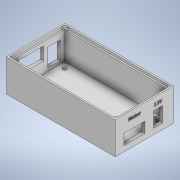
# Autodesk Inventor part: Caixa plaquinha valvulav2
Saved by Autodesk Inventor 2020 (Build 240168000, 168)
## iProperties
Created: 2022-10-16
Part Number: Caixa plaquinha valvulav2
Material: Genérico
Document SubType Name: Modeling
Designer: Gabriel
Density: 1 g/cm^3
Appearance: Padrão
Author: Gabriel
Autodesk Inventor part; units mm, degrees
ref_plane "YZ Plane" through (0, 0, 0) normal (1, 0, 0) x (0, 1, 0)
ref_plane "XZ Plane" through (0, 0, 0) normal (0, 1, 0) x (-1, 0, 0)
ref_plane "XY Plane" through (0, 0, 0) normal (0, 0, 1) x (1, 0, 0)
sketch "Esboço1" plane through (0, 0, 0) normal (0, 1, 0) x (-1, 0, 0)
  line L0 (62.5795, 27.2159) -> (-45.4205, 27.2159)
  line L1 (-45.4205, 27.2159) -> (-45.4205, -30.7841)
  line L2 (-45.4205, -30.7841) -> (62.5795, -30.7841)
  line L3 (62.5795, -30.7841) -> (62.5795, 27.2159)
  point P0 (0, 0)
  dimension "d0" = 58
  dimension "d1" = 108
  constraints: 8 end point, 2 parallel, 1 horizontal, 1 perpendicular
  measures "d0" distance between parallel lines of L2 L0
  measures "d1" distance of L1.end L2.end
extrude "Extrusão1" add sketch "Esboço1" along normal blind 32
sketch "Esboço2" plane through (0, 32, 0) normal (0, 1, 0) x (1, 0, 0)
  line L0 (-59.5795, 27.7841) -> (42.4205, 27.7841)
  line L1 (42.4205, 27.7841) -> (42.4205, -24.2159)
  line L2 (42.4205, -24.2159) -> (-59.5795, -24.2159)
  line L3 (-59.5795, -24.2159) -> (-59.5795, 27.7841)
  line L4 (-62.5795, 30.7841) -> (-62.5795, -27.2159) projected
  line L5 (45.4205, 30.7841) -> (-62.5795, 30.7841) projected
  point P0 (0, 0)
  dimension "d4" = 3
  dimension "d5" = 102
  dimension "d6" = 3
  dimension "d7" = 52
  constraints: 8 end point, 2 parallel, 1 horizontal, 1 perpendicular
  measures "d4" distance between parallel lines of L4 L3
  measures "d5" distance between parallel lines of L1 L3
  measures "d6" distance between parallel lines of L5 L0
  measures "d7" distance between parallel lines of L0 L2
extrude "Extrusão2" cut sketch "Esboço2" against normal blind 30
sketch "Esboço4" plane through (0, 32, 0) normal (0, 1, 0) x (1, 0, 0)
  line L0 (-61.0795, 29.2841) -> (43.9205, 29.2841)
  line L1 (43.9205, 29.2841) -> (43.9205, -25.7159)
  line L2 (43.9205, -25.7159) -> (-61.0795, -25.7159)
  line L3 (-61.0795, -25.7159) -> (-61.0795, 29.2841)
  line L4 (45.4205, 30.7841) -> (-62.5795, 30.7841) projected
  line L5 (-62.5795, 30.7841) -> (-62.5795, -27.2159) projected
  line L6 (-62.5795, -27.2159) -> (45.4205, -27.2159) projected
  line L7 (45.4205, -27.2159) -> (45.4205, 30.7841) projected
  point P0 (0, 0)
  dimension "d10" = 1.5
  dimension "d11" = 1.5
  dimension "d12" = 1.5
  dimension "d13" = 1.5
  constraints: 8 end point, 2 parallel, 1 horizontal, 1 perpendicular
  measures "d10" distance between parallel lines of L4 L0
  measures "d11" distance between parallel lines of L5 L3
  measures "d12" distance between parallel lines of L6 L2
  measures "d13" distance between parallel lines of L7 L1
extrude "Extrusão3" cut sketch "Esboço4" against normal blind 2.5 contours L0 L1 L2 L3
sketch "Esboço5" plane through (42.4205, 2, -27.7841) normal (-1, 0, 0) x (0, 0, 1)
  line L0 (0, 0) -> (52, 0) projected
  line L1 (8.1, 3.75) -> (17.1, 3.75)
  line L2 (17.1, 3.75) -> (17.1, 18.75)
  line L3 (17.1, 18.75) -> (8.1, 18.75)
  line L4 (8.1, 18.75) -> (8.1, 3.75)
  line L5 (46.3, 3.5) -> (25.6, 3.5)
  line L6 (25.6, 3.5) -> (25.6, 14)
  line L7 (25.6, 14) -> (46.3, 14)
  line L8 (46.3, 14) -> (46.3, 3.5)
  line L9 (52, 27.5) -> (0, 27.5) projected
  point P0 (27.7841, -2)
  point P1 (25.6, 0)
  point P2 (17.1, 0)
  dimension "d17" = 9
  dimension "d20" = 20.7
  dimension "d23" = 8.5
  dimension "d24" = 8.1
  dimension "d25" = 5.7
  dimension "d55" = 3.75
  dimension "d56" = 15
  dimension "d57" = 3.5
  dimension "d58" = 10.5
  constraints: 16 end point, 4 parallel, 2 horizontal, 2 perpendicular
  measures "d17" distance between parallel lines of L2 L4
  measures "d20" distance between parallel lines of L6 L8
  measures "d23" distance between parallel lines of L6 L2
  measures "d24" distance from line of L9.end L4
  measures "d25" distance from line of L9.start L8
  measures "d55" distance between parallel lines of L1 L0
  measures "d56" distance between parallel lines of L3 L1
  measures "d57" distance between parallel lines of L0 L5
  measures "d58" distance between parallel lines of L7 L5
extrude "Extrusão4" cut sketch "Esboço5" against normal blind 5
sketch "Esboço6" plane through (0, 2, 0) normal (0, 1, 0) x (1, 0, 0)
  line L0 (45.4205, 2.1841) -> (45.4205, -18.5159) projected
  line L1 (42.4205, 27.7841) -> (42.4205, -24.2159) projected
  line L2 (45.4205, -18.5159) -> (42.4205, -18.5159)
  line L3 (42.4205, -18.5159) -> (42.4205, 2.1841)
  line L4 (42.4205, 2.1841) -> (45.4205, 2.1841)
  line L5 (45.4205, 2.1841) -> (45.4205, -18.5159)
  line L6 (45.4205, 19.6841) -> (45.4205, 10.6841) projected
  line L7 (45.4205, 19.6841) -> (42.4205, 19.6841)
  line L8 (42.4205, 19.6841) -> (42.4205, 10.6841)
  line L9 (42.4205, 10.6841) -> (45.4205, 10.6841)
  line L10 (45.4205, 10.6841) -> (45.4205, 19.6841)
  point P0 (0, 0)
  point P1 (42.4205, 10.6841)
  constraints: 16 end point, 4 parallel, 2 horizontal, 2 perpendicular, 1 point on line
extrude "Extrusão5" add sketch "Esboço6" along normal blind 1
sketch "Esboço7" plane through (-59.5795, 2, 24.2159) normal (1, 0, 0) x (0, 0, -1)
  line L0 (47.5, 3) -> (35, 3)
  line L1 (35, 3) -> (35, 21)
  line L2 (35, 21) -> (47.5, 21)
  line L3 (47.5, 21) -> (47.5, 3)
  line L4 (6, 11) -> (31, 11)
  line L5 (31, 11) -> (31, 24)
  line L6 (31, 24) -> (6, 24)
  line L7 (6, 24) -> (6, 11)
  line L8 (0, 0) -> (52, 0) projected
  point P0 (24.2159, -2)
  point P1 (52, 27.5)
  point P2 (0, 27.5)
  dimension "d31" = 4.5
  dimension "d32" = 12.5
  dimension "d33" = 6
  dimension "d34" = 25
  dimension "d35" = 13
  dimension "d36" = 11
  dimension "d39" = 18
  dimension "d59" = 3
  constraints: 16 end point, 4 parallel, 2 horizontal, 2 perpendicular
  measures "d31" distance from line of L3 point (52, 27.5)
  measures "d32" distance between parallel lines of L3 L1
  measures "d33" distance from line of point (0, 27.5) L7
  measures "d34" distance between parallel lines of L5 L7
  measures "d35" distance between parallel lines of L6 L4
  measures "d36" distance between parallel lines of L8 L4
  measures "d39" distance between parallel lines of L0 L2
  measures "d59" distance between parallel lines of L8 L0
extrude "Extrusão6" cut sketch "Esboço7" against normal blind 5
sketch "Esboço9" plane through (0, 2, 0) normal (0, 1, 0) x (1, 0, 0)
  line L0 (42.4205, -24.2159) -> (-59.5795, -24.2159) projected
  line L1 (5.9205, -24.2159) -> (10.9205, -24.2159)
  line L2 (10.9205, -24.2159) -> (10.9205, -27.2159)
  line L3 (10.9205, -27.2159) -> (5.9205, -27.2159)
  line L4 (5.9205, -27.2159) -> (5.9205, -24.2159)
  line L5 (10.9205, -27.2159) -> (5.9205, -27.2159) projected
  point P0 (0, 0)
  dimension "d50" = 0
  constraints: 8 end point, 2 parallel, 1 horizontal, 1 perpendicular
  measures "d50" distance between parallel lines of L5 L3
extrude "Extrusão8" add sketch "Esboço9" along normal blind 1
sketch "Esboço10" plane through (45.4205, 0, 27.2159) normal (1, 0, 0) x (0, 0, -1)
  line L0 (36.0799, 28.5533) -> (48.8276, 28.5533) construction
  line L1 (48.8276, 28.5533) -> (48.8276, 22.0035) construction
  line L2 (48.8276, 22.0035) -> (36.0799, 22.0035) construction
  line L3 (36.0799, 22.0035) -> (36.0799, 28.5533) construction
  line L4 (13.7499, 26.9393) -> (24.4451, 26.9393) construction
  line L5 (24.4451, 26.9393) -> (24.4451, 23.827) construction
  line L6 (24.4451, 23.827) -> (13.7499, 23.827) construction
  line L7 (13.7499, 23.827) -> (13.7499, 26.9393) construction
  line L8 (16.286, 23.8893) -> (15.5247, 23.8893)
  line L9 (15.5247, 23.8893) -> (15.5247, 25.9111)
  line L10 (15.5247, 25.9111) -> (14.9711, 24.606)
  line L11 (14.9711, 24.606) -> (14.4471, 24.606)
  line L12 (14.4471, 24.606) -> (13.8935, 25.9111)
  line L13 (13.8935, 25.9111) -> (13.8935, 23.8893)
  line L14 (13.8935, 23.8893) -> (13.1717, 23.8893)
  line L15 (13.1717, 23.8893) -> (13.1717, 26.9393)
  line L16 (13.1717, 26.9393) -> (14.0541, 26.9393)
  line L17 (14.0541, 26.9393) -> (14.7313, 25.434)
  line L18 (14.7313, 25.434) -> (15.4036, 26.9393)
  line L19 (15.4036, 26.9393) -> (16.286, 26.9393)
  line L20 (16.286, 26.9393) -> (16.286, 23.8893)
  spline S0 degree 2 poles (19.0839, 25.0386) (19.0839, 24.4701) (18.4635, 23.8176) (17.8975, 23.8176) knots 0 0 0 1 2 2 2
  spline S1 degree 2 poles (17.8975, 23.8176) (17.334, 23.8176) (16.7087, 24.4701) (16.7087, 25.0386) knots 0 0 0 1 2 2 2
  spline S2 degree 2 poles (16.7087, 25.0386) (16.7087, 25.612) (17.334, 26.262) (17.8975, 26.262) knots 0 0 0 1 2 2 2
  spline S3 degree 2 poles (17.8975, 26.262) (18.461, 26.262) (19.0839, 25.6095) (19.0839, 25.0386) knots 0 0 0 1 2 2 2
  spline S4 degree 2 poles (18.3498, 25.0336) (18.3498, 25.2388) (18.2831, 25.5131) (18.2238, 25.5947) knots 0 0 0 1 2 2 2
  spline S5 degree 2 poles (18.2238, 25.5947) (18.1595, 25.6812) (17.9989, 25.7479) (17.8975, 25.7479) knots 0 0 0 1 2 2 2
  spline S6 degree 2 poles (17.8975, 25.7479) (17.7986, 25.7479) (17.6429, 25.6886) (17.5787, 25.6046) knots 0 0 0 1 2 2 2
  spline S7 degree 2 poles (17.5787, 25.6046) (17.5169, 25.5255) (17.4427, 25.2462) (17.4427, 25.0336) knots 0 0 0 1 2 2 2
  spline S8 degree 2 poles (17.4427, 25.0336) (17.4427, 24.8235) (17.5119, 24.564) (17.5688, 24.4849) knots 0 0 0 1 2 2 2
  spline S9 degree 2 poles (17.5688, 24.4849) (17.6256, 24.4058) (17.7986, 24.3317) (17.9025, 24.3317) knots 0 0 0 1 2 2 2
  spline S10 degree 2 poles (17.9025, 24.3317) (17.989, 24.3317) (18.1669, 24.4058) (18.2213, 24.48) knots 0 0 0 1 2 2 2
  spline S11 degree 2 poles (18.2213, 24.48) (18.2831, 24.5665) (18.3498, 24.8161) (18.3498, 25.0336) knots 0 0 0 1 2 2 2
  spline S12 degree 2 poles (20.3444, 23.8448) (19.907, 23.8448) (19.5065, 24.2056) (19.5065, 24.6159) knots 0 0 0 1 2 2 2
  line L21 (19.5065, 24.6159) -> (19.5065, 25.6911)
  line L22 (19.5065, 25.6911) -> (19.2322, 25.6911)
  line L23 (19.2322, 25.6911) -> (19.2322, 26.1904)
  line L24 (19.2322, 26.1904) -> (19.5065, 26.1904)
  line L25 (19.5065, 26.1904) -> (19.5065, 26.8478)
  line L26 (19.5065, 26.8478) -> (20.2233, 26.8478)
  line L27 (20.2233, 26.8478) -> (20.2233, 26.1904)
  line L28 (20.2233, 26.1904) -> (20.9154, 26.1904)
  line L29 (20.9154, 26.1904) -> (20.9154, 25.6911)
  line L30 (20.9154, 25.6911) -> (20.2233, 25.6911)
  line L31 (20.2233, 25.6911) -> (20.2233, 24.873)
  spline S13 degree 2 poles (20.2233, 24.873) (20.2233, 24.7519) (20.2283, 24.5714) (20.2579, 24.4998) knots 0 0 0 1 2 2 2
  spline S14 degree 2 poles (20.2579, 24.4998) (20.2876, 24.4281) (20.4334, 24.344) (20.5718, 24.344) knots 0 0 0 1 2 2 2
  spline S15 degree 2 poles (20.5718, 24.344) (20.6311, 24.344) (20.8165, 24.3935) (20.8536, 24.4132) knots 0 0 0 1 2 2 2
  line L32 (20.8536, 24.4132) -> (20.9154, 24.4132)
  line L33 (20.9154, 24.4132) -> (20.9154, 23.909)
  spline S16 degree 2 poles (20.9154, 23.909) (20.7992, 23.8794) (20.5372, 23.8448) (20.3444, 23.8448) knots 0 0 0 1 2 2 2
  spline S17 degree 2 poles (23.4142, 25.0386) (23.4142, 24.4701) (22.7938, 23.8176) (22.2278, 23.8176) knots 0 0 0 1 2 2 2
  spline S18 degree 2 poles (22.2278, 23.8176) (21.6643, 23.8176) (21.039, 24.4701) (21.039, 25.0386) knots 0 0 0 1 2 2 2
  spline S19 degree 2 poles (21.039, 25.0386) (21.039, 25.612) (21.6643, 26.262) (22.2278, 26.262) knots 0 0 0 1 2 2 2
  spline S20 degree 2 poles (22.2278, 26.262) (22.7914, 26.262) (23.4142, 25.6095) (23.4142, 25.0386) knots 0 0 0 1 2 2 2
  spline S21 degree 2 poles (22.6801, 25.0336) (22.6801, 25.2388) (22.6134, 25.5131) (22.5541, 25.5947) knots 0 0 0 1 2 2 2
  spline S22 degree 2 poles (22.5541, 25.5947) (22.4898, 25.6812) (22.3292, 25.7479) (22.2278, 25.7479) knots 0 0 0 1 2 2 2
  spline S23 degree 2 poles (22.2278, 25.7479) (22.129, 25.7479) (21.9732, 25.6886) (21.909, 25.6046) knots 0 0 0 1 2 2 2
  spline S24 degree 2 poles (21.909, 25.6046) (21.8472, 25.5255) (21.773, 25.2462) (21.773, 25.0336) knots 0 0 0 1 2 2 2
  spline S25 degree 2 poles (21.773, 25.0336) (21.773, 24.8235) (21.8422, 24.564) (21.8991, 24.4849) knots 0 0 0 1 2 2 2
  spline S26 degree 2 poles (21.8991, 24.4849) (21.9559, 24.4058) (22.129, 24.3317) (22.2328, 24.3317) knots 0 0 0 1 2 2 2
  spline S27 degree 2 poles (22.2328, 24.3317) (22.3193, 24.3317) (22.4972, 24.4058) (22.5516, 24.48) knots 0 0 0 1 2 2 2
  spline S28 degree 2 poles (22.5516, 24.48) (22.6134, 24.5665) (22.6801, 24.8161) (22.6801, 25.0336) knots 0 0 0 1 2 2 2
  line L34 (25.3396, 25.5106) -> (25.2803, 25.5106)
  spline S29 degree 2 poles (25.2803, 25.5106) (25.2383, 25.5255) (25.0826, 25.5403) (24.9886, 25.5403) knots 0 0 0 1 2 2 2
  spline S30 degree 2 poles (24.9886, 25.5403) (24.8774, 25.5403) (24.6278, 25.4736) (24.5116, 25.4291) knots 0 0 0 1 2 2 2
  line L35 (24.5116, 25.4291) -> (24.5116, 23.8893)
  line L36 (24.5116, 23.8893) -> (23.7948, 23.8893)
  line L37 (23.7948, 23.8893) -> (23.7948, 26.1904)
  line L38 (23.7948, 26.1904) -> (24.5116, 26.1904)
  line L39 (24.5116, 26.1904) -> (24.5116, 25.8592)
  spline S31 degree 2 poles (24.5116, 25.8592) (24.561, 25.9036) (24.7341, 26.0421) (24.8057, 26.0841) knots 0 0 0 1 2 2 2
  spline S32 degree 2 poles (24.8057, 26.0841) (24.8848, 26.131) (25.0924, 26.1978) (25.1839, 26.1978) knots 0 0 0 1 2 2 2
  spline S33 degree 2 poles (25.1839, 26.1978) (25.2185, 26.1978) (25.305, 26.1928) (25.3396, 26.1904) knots 0 0 0 1 2 2 2
  line L40 (25.3396, 26.1904) -> (25.3396, 25.5106)
  line L41 (40.7496, 23.7237) -> (38.7352, 23.7237)
  line L42 (38.7352, 23.7237) -> (38.7352, 24.2551)
  line L43 (38.7352, 24.2551) -> (39.3778, 24.2551)
  line L44 (39.3778, 24.2551) -> (39.3778, 25.8691)
  line L45 (39.3778, 25.8691) -> (38.7352, 25.8691)
  line L46 (38.7352, 25.8691) -> (38.7352, 26.3659)
  spline S34 degree 2 poles (38.7352, 26.3659) (38.8761, 26.3659) (39.1554, 26.403) (39.2394, 26.4425) knots 0 0 0 1 2 2 2
  spline S35 degree 2 poles (39.2394, 26.4425) (39.3358, 26.492) (39.4445, 26.6576) (39.4544, 26.7811) knots 0 0 0 1 2 2 2
  line L47 (39.4544, 26.7811) -> (40.1218, 26.7811)
  line L48 (40.1218, 26.7811) -> (40.1218, 24.2551)
  line L49 (40.1218, 24.2551) -> (40.7496, 24.2551)
  line L50 (40.7496, 24.2551) -> (40.7496, 23.7237)
  line L51 (43.5573, 23.7237) -> (41.3156, 23.7237)
  line L52 (41.3156, 23.7237) -> (41.3156, 24.2205)
  spline S36 degree 2 poles (41.3156, 24.2205) (41.5998, 24.4479) (42.0546, 24.8483) (42.2251, 25.0288) knots 0 0 0 1 2 2 2
  spline S37 degree 2 poles (42.2251, 25.0288) (42.45, 25.2636) (42.6502, 25.6219) (42.6502, 25.8098) knots 0 0 0 1 2 2 2
  spline S38 degree 2 poles (42.6502, 25.8098) (42.6502, 26.0224) (42.3957, 26.2497) (42.1683, 26.2497) knots 0 0 0 1 2 2 2
  spline S39 degree 2 poles (42.1683, 26.2497) (42.0521, 26.2497) (41.8445, 26.1929) (41.7382, 26.1484) knots 0 0 0 1 2 2 2
  spline S40 degree 2 poles (41.7382, 26.1484) (41.6344, 26.1014) (41.4861, 26.0026) (41.449, 25.9779) knots 0 0 0 1 2 2 2
  line L53 (41.449, 25.9779) -> (41.3897, 25.9779)
  line L54 (41.3897, 25.9779) -> (41.3897, 26.6427)
  spline S41 degree 2 poles (41.3897, 26.6427) (41.5182, 26.7045) (42.0669, 26.833) (42.3215, 26.833) knots 0 0 0 1 2 2 2
  spline S42 degree 2 poles (42.3215, 26.833) (42.8653, 26.833) (43.4239, 26.3486) (43.4239, 25.9111) knots 0 0 0 1 2 2 2
  spline S43 degree 2 poles (43.4239, 25.9111) (43.4239, 25.6417) (43.1693, 25.1227) (42.8752, 24.8261) knots 0 0 0 1 2 2 2
  spline S44 degree 2 poles (42.8752, 24.8261) (42.6898, 24.6432) (42.3413, 24.3589) (42.2647, 24.2996) knots 0 0 0 1 2 2 2
  line L55 (42.2647, 24.2996) -> (43.5573, 24.2996)
  line L56 (43.5573, 24.2996) -> (43.5573, 23.7237)
  line L57 (46.5406, 26.7737) -> (45.4926, 23.7237)
  line L58 (45.4926, 23.7237) -> (44.6943, 23.7237)
  line L59 (44.6943, 23.7237) -> (43.6463, 26.7737)
  line L60 (43.6463, 26.7737) -> (44.4397, 26.7737)
  line L61 (44.4397, 26.7737) -> (45.1046, 24.705)
  line L62 (45.1046, 24.705) -> (45.767, 26.7737)
  line L63 (45.767, 26.7737) -> (46.5406, 26.7737)
  point P0 (27.2159, 0)
  constraints: 4 other
extrude "Extrusão9" cut sketch "Esboço10" against normal blind 0.8
sketch "Esboço11" plane through (-62.5795, 0, -30.7841) normal (-1, 0, 0) x (0, 0, 1)
  line L0 (32.154, 11.2221) -> (40.856, 11.2221) construction
  line L1 (40.856, 11.2221) -> (40.856, 8.0726) construction
  line L2 (40.856, 8.0726) -> (32.154, 8.0726) construction
  line L3 (32.154, 8.0726) -> (32.154, 11.2221) construction
  line L4 (7.8779, 28.5473) -> (19.6465, 28.5473) construction
  line L5 (19.6465, 28.5473) -> (19.6465, 24.5765) construction
  line L6 (19.6465, 24.5765) -> (7.8779, 24.5765) construction
  line L7 (7.8779, 24.5765) -> (7.8779, 28.5473) construction
  line L8 (8.874, 26.9175) -> (7.8103, 26.9175)
  line L9 (7.8103, 26.9175) -> (7.8103, 27.2265)
  line L10 (7.8103, 27.2265) -> (8.874, 27.2265)
  line L11 (8.874, 27.2265) -> (8.874, 26.9175)
  spline S0 degree 2 poles (12.5502, 26.6874) (12.5502, 26.5381) (12.4113, 26.2478) (12.2869, 26.1483) knots 0 0 0 1 2 2 2
  spline S1 degree 2 poles (12.2869, 26.1483) (12.1501, 26.0384) (11.7872, 25.916) (11.5322, 25.916) knots 0 0 0 1 2 2 2
  spline S2 degree 2 poles (11.5322, 25.916) (11.2564, 25.916) (10.8168, 26.0176) (10.5908, 26.1192) knots 0 0 0 1 2 2 2
  line L12 (10.5908, 26.1192) -> (10.5908, 26.5422)
  line L13 (10.5908, 26.5422) -> (10.6157, 26.5422)
  spline S3 degree 2 poles (10.6157, 26.5422) (10.8085, 26.3826) (11.3124, 26.2084) (11.5363, 26.2084) knots 0 0 0 1 2 2 2
  spline S4 degree 2 poles (11.5363, 26.2084) (11.8494, 26.2084) (12.1998, 26.4427) (12.1998, 26.6397) knots 0 0 0 1 2 2 2
  spline S5 degree 2 poles (12.1998, 26.6397) (12.1998, 26.8076) (12.0339, 26.9673) (11.8639, 27.0129) knots 0 0 0 1 2 2 2
  spline S6 degree 2 poles (11.8639, 27.0129) (11.7374, 27.0461) (11.4368, 27.0917) (11.2709, 27.1249) knots 0 0 0 1 2 2 2
  spline S7 degree 2 poles (11.2709, 27.1249) (10.9309, 27.1974) (10.6053, 27.5437) (10.6053, 27.8216) knots 0 0 0 1 2 2 2
  spline S8 degree 2 poles (10.6053, 27.8216) (10.6053, 28.1388) (11.1444, 28.5473) (11.5612, 28.5473) knots 0 0 0 1 2 2 2
  spline S9 degree 2 poles (11.5612, 28.5473) (11.8287, 28.5473) (12.2765, 28.4457) (12.4486, 28.369) knots 0 0 0 1 2 2 2
  line L14 (12.4486, 28.369) -> (12.4486, 27.9708)
  line L15 (12.4486, 27.9708) -> (12.4238, 27.9708)
  spline S10 degree 2 poles (12.4238, 27.9708) (12.2786, 28.0932) (11.8059, 28.2549) (11.5571, 28.2549) knots 0 0 0 1 2 2 2
  spline S11 degree 2 poles (11.5571, 28.2549) (11.2854, 28.2549) (10.9557, 28.031) (10.9557, 27.8527) knots 0 0 0 1 2 2 2
  spline S12 degree 2 poles (10.9557, 27.8527) (10.9557, 27.6951) (11.1195, 27.5147) (11.3269, 27.467) knots 0 0 0 1 2 2 2
  spline S13 degree 2 poles (11.3269, 27.467) (11.4368, 27.4421) (11.839, 27.3737) (11.98, 27.3384) knots 0 0 0 1 2 2 2
  spline S14 degree 2 poles (11.98, 27.3384) (12.2641, 27.2638) (12.5502, 26.959) (12.5502, 26.6874) knots 0 0 0 1 2 2 2
  line L16 (13.3921, 25.9617) -> (13.0707, 25.9617)
  line L17 (13.0707, 25.9617) -> (13.0707, 27.8672)
  line L18 (13.0707, 27.8672) -> (13.3921, 27.8672)
  line L19 (13.3921, 27.8672) -> (13.3921, 25.9617)
  line L20 (13.4128, 28.1865) -> (13.0499, 28.1865)
  line L21 (13.0499, 28.1865) -> (13.0499, 28.5182)
  line L22 (13.0499, 28.5182) -> (13.4128, 28.5182)
  line L23 (13.4128, 28.5182) -> (13.4128, 28.1865)
  spline S15 degree 2 poles (15.5734, 26.1794) (15.5734, 25.6942) (15.1338, 25.2401) (14.6755, 25.2401) knots 0 0 0 1 2 2 2
  spline S16 degree 2 poles (14.6755, 25.2401) (14.5242, 25.2401) (14.236, 25.2836) (14.095, 25.321) knots 0 0 0 1 2 2 2
  line L24 (14.095, 25.321) -> (14.095, 25.6486)
  line L25 (14.095, 25.6486) -> (14.1116, 25.6486)
  spline S17 degree 2 poles (14.1116, 25.6486) (14.1904, 25.6175) (14.5325, 25.5283) (14.7025, 25.5283) knots 0 0 0 1 2 2 2
  spline S18 degree 2 poles (14.7025, 25.5283) (14.8663, 25.5283) (15.0819, 25.6071) (15.1421, 25.6755) knots 0 0 0 1 2 2 2
  spline S19 degree 2 poles (15.1421, 25.6755) (15.2001, 25.7419) (15.252, 25.9306) (15.252, 26.0467) knots 0 0 0 1 2 2 2
  line L26 (15.252, 26.0467) -> (15.252, 26.2188)
  spline S20 degree 2 poles (15.252, 26.2188) (15.1068, 26.1026) (14.8435, 25.9886) (14.6382, 25.9886) knots 0 0 0 1 2 2 2
  spline S21 degree 2 poles (14.6382, 25.9886) (14.2961, 25.9886) (13.8959, 26.4821) (13.8959, 26.932) knots 0 0 0 1 2 2 2
  spline S22 degree 2 poles (13.8959, 26.932) (13.8959, 27.1788) (14.0348, 27.5354) (14.153, 27.664) knots 0 0 0 1 2 2 2
  spline S23 degree 2 poles (14.153, 27.664) (14.265, 27.7863) (14.5822, 27.9211) (14.7378, 27.9211) knots 0 0 0 1 2 2 2
  spline S24 degree 2 poles (14.7378, 27.9211) (14.9036, 27.9211) (15.1276, 27.8547) (15.252, 27.7863) knots 0 0 0 1 2 2 2
  line L27 (15.252, 27.7863) -> (15.2727, 27.8672)
  line L28 (15.2727, 27.8672) -> (15.5734, 27.8672)
  line L29 (15.5734, 27.8672) -> (15.5734, 26.1794)
  line L30 (15.252, 26.4842) -> (15.252, 27.525)
  spline S25 degree 2 poles (15.252, 27.525) (15.1234, 27.5831) (14.9036, 27.6329) (14.7958, 27.6329) knots 0 0 0 1 2 2 2
  spline S26 degree 2 poles (14.7958, 27.6329) (14.5304, 27.6329) (14.2277, 27.2762) (14.2277, 26.9383) knots 0 0 0 1 2 2 2
  spline S27 degree 2 poles (14.2277, 26.9383) (14.2277, 26.6169) (14.4537, 26.2851) (14.7129, 26.2851) knots 0 0 0 1 2 2 2
  spline S28 degree 2 poles (14.7129, 26.2851) (14.8539, 26.2851) (15.1338, 26.3929) (15.252, 26.4842) knots 0 0 0 1 2 2 2
  line L31 (19.6166, 26.9362) -> (18.6877, 26.9362)
  line L32 (18.6877, 26.9362) -> (18.6877, 26.0073)
  line L33 (18.6877, 26.0073) -> (18.4036, 26.0073)
  line L34 (18.4036, 26.0073) -> (18.4036, 26.9362)
  line L35 (18.4036, 26.9362) -> (17.4747, 26.9362)
  line L36 (17.4747, 26.9362) -> (17.4747, 27.2099)
  line L37 (17.4747, 27.2099) -> (18.4036, 27.2099)
  line L38 (18.4036, 27.2099) -> (18.4036, 28.1388)
  line L39 (18.4036, 28.1388) -> (18.6877, 28.1388)
  line L40 (18.6877, 28.1388) -> (18.6877, 27.2099)
  line L41 (18.6877, 27.2099) -> (19.6166, 27.2099)
  line L42 (19.6166, 27.2099) -> (19.6166, 26.9362)
  spline S29 degree 2 poles (33.738, 8.0535) (33.1226, 8.0535) (32.4602, 8.6467) (32.4602, 9.2201) knots 0 0 0 1 2 2 2
  line L43 (32.4602, 9.2201) -> (32.4602, 11.1677)
  line L44 (32.4602, 11.1677) -> (33.2264, 11.1677)
  line L45 (33.2264, 11.1677) -> (33.2264, 9.2646)
  spline S30 degree 2 poles (33.2264, 9.2646) (33.2264, 8.9457) (33.4661, 8.6343) (33.738, 8.6343) knots 0 0 0 1 2 2 2
  spline S31 degree 2 poles (33.738, 8.6343) (34.0025, 8.6343) (34.2496, 8.9334) (34.2496, 9.2646) knots 0 0 0 1 2 2 2
  line L46 (34.2496, 9.2646) -> (34.2496, 11.1677)
  line L47 (34.2496, 11.1677) -> (35.0158, 11.1677)
  line L48 (35.0158, 11.1677) -> (35.0158, 9.2225)
  spline S32 degree 2 poles (35.0158, 9.2225) (35.0158, 8.659) (34.3708, 8.0535) (33.738, 8.0535) knots 0 0 0 1 2 2 2
  spline S33 degree 2 poles (36.5458, 8.0634) (36.1948, 8.0634) (35.6659, 8.1993) (35.4385, 8.2982) knots 0 0 0 1 2 2 2
  line L49 (35.4385, 8.2982) -> (35.4385, 9.0248)
  line L50 (35.4385, 9.0248) -> (35.5077, 9.0248)
  spline S34 degree 2 poles (35.5077, 9.0248) (35.7376, 8.8296) (36.2887, 8.6195) (36.5483, 8.6195) knots 0 0 0 1 2 2 2
  spline S35 degree 2 poles (36.5483, 8.6195) (36.615, 8.6195) (36.83, 8.6491) (36.8943, 8.6788) knots 0 0 0 1 2 2 2
  spline S36 degree 2 poles (36.8943, 8.6788) (36.9734, 8.7134) (37.0846, 8.8394) (37.0846, 8.9408) knots 0 0 0 1 2 2 2
  spline S37 degree 2 poles (37.0846, 8.9408) (37.0846, 9.0569) (36.9042, 9.2003) (36.7806, 9.2324) knots 0 0 0 1 2 2 2
  spline S38 degree 2 poles (36.7806, 9.2324) (36.6249, 9.2745) (36.2714, 9.3461) (36.1157, 9.4005) knots 0 0 0 1 2 2 2
  spline S39 degree 2 poles (36.1157, 9.4005) (35.7623, 9.5241) (35.4558, 9.9467) (35.4558, 10.2631) knots 0 0 0 1 2 2 2
  spline S40 degree 2 poles (35.4558, 10.2631) (35.4558, 10.6907) (36.18, 11.2221) (36.7237, 11.2221) knots 0 0 0 1 2 2 2
  spline S41 degree 2 poles (36.7237, 11.2221) (36.9956, 11.2221) (37.5344, 11.1109) (37.747, 11.017) knots 0 0 0 1 2 2 2
  line L51 (37.747, 11.017) -> (37.747, 10.32)
  line L52 (37.747, 10.32) -> (37.6803, 10.32)
  spline S42 degree 2 poles (37.6803, 10.32) (37.5097, 10.4658) (37.0203, 10.666) (36.7633, 10.666) knots 0 0 0 1 2 2 2
  spline S43 degree 2 poles (36.7633, 10.666) (36.662, 10.666) (36.5038, 10.6363) (36.4148, 10.5968) knots 0 0 0 1 2 2 2
  spline S44 degree 2 poles (36.4148, 10.5968) (36.3431, 10.5646) (36.2393, 10.4361) (36.2393, 10.357) knots 0 0 0 1 2 2 2
  spline S45 degree 2 poles (36.2393, 10.357) (36.2393, 10.2384) (36.4049, 10.1025) (36.6422, 10.0481) knots 0 0 0 1 2 2 2
  spline S46 degree 2 poles (36.6422, 10.0481) (36.7954, 10.0135) (37.0797, 9.9467) (37.2428, 9.8899) knots 0 0 0 1 2 2 2
  spline S47 degree 2 poles (37.2428, 9.8899) (37.5592, 9.7737) (37.8681, 9.3881) (37.8681, 9.0718) knots 0 0 0 1 2 2 2
  spline S48 degree 2 poles (37.8681, 9.0718) (37.8681, 8.617) (37.1538, 8.0634) (36.5458, 8.0634) knots 0 0 0 1 2 2 2
  spline S49 degree 2 poles (40.6981, 9.052) (40.6981, 8.8246) (40.5251, 8.4811) (40.3818, 8.3674) knots 0 0 0 1 2 2 2
  spline S50 degree 2 poles (40.3818, 8.3674) (40.2088, 8.2314) (39.7985, 8.1177) (39.4796, 8.1177) knots 0 0 0 1 2 2 2
  line L53 (39.4796, 8.1177) -> (38.2611, 8.1177)
  line L54 (38.2611, 8.1177) -> (38.2611, 11.1677)
  line L55 (38.2611, 11.1677) -> (39.3363, 11.1677)
  spline S51 degree 2 poles (39.3363, 11.1677) (39.6724, 11.1677) (40.0184, 11.1158) (40.1692, 11.0343) knots 0 0 0 1 2 2 2
  spline S52 degree 2 poles (40.1692, 11.0343) (40.3348, 10.9478) (40.4955, 10.6512) (40.4955, 10.4584) knots 0 0 0 1 2 2 2
  spline S53 degree 2 poles (40.4955, 10.4584) (40.4955, 10.2359) (40.273, 9.8874) (40.0753, 9.8059) knots 0 0 0 1 2 2 2
  line L56 (40.0753, 9.8059) -> (40.0753, 9.791)
  spline S54 degree 2 poles (40.0753, 9.791) (40.3595, 9.7317) (40.6981, 9.3634) (40.6981, 9.052) knots 0 0 0 1 2 2 2
  spline S55 degree 2 poles (39.9072, 9.0644) (39.9072, 9.2077) (39.7935, 9.3684) (39.6798, 9.4104) knots 0 0 0 1 2 2 2
  spline S56 degree 2 poles (39.6798, 9.4104) (39.6106, 9.4376) (39.3659, 9.4425) (39.1633, 9.4425) knots 0 0 0 1 2 2 2
  line L57 (39.1633, 9.4425) -> (39.0224, 9.4425)
  line L58 (39.0224, 9.4425) -> (39.0224, 8.6738)
  line L59 (39.0224, 8.6738) -> (39.0644, 8.6738)
  spline S57 degree 2 poles (39.0644, 8.6738) (39.361, 8.6738) (39.5884, 8.6813) (39.707, 8.7332) knots 0 0 0 1 2 2 2
  spline S58 degree 2 poles (39.707, 8.7332) (39.8108, 8.7801) (39.9072, 8.9531) (39.9072, 9.0644) knots 0 0 0 1 2 2 2
  spline S59 degree 2 poles (39.7169, 10.3076) (39.7169, 10.3817) (39.6403, 10.5375) (39.5612, 10.5721) knots 0 0 0 1 2 2 2
  spline S60 degree 2 poles (39.5612, 10.5721) (39.487, 10.6067) (39.2794, 10.6116) (39.0743, 10.6116) knots 0 0 0 1 2 2 2
  line L60 (39.0743, 10.6116) -> (39.0224, 10.6116)
  line L61 (39.0224, 10.6116) -> (39.0224, 9.964)
  line L62 (39.0224, 9.964) -> (39.1188, 9.964)
  spline S61 degree 2 poles (39.1188, 9.964) (39.314, 9.964) (39.4722, 9.9715) (39.5562, 10.011) knots 0 0 0 1 2 2 2
  spline S62 degree 2 poles (39.5562, 10.011) (39.6477, 10.0555) (39.7169, 10.2063) (39.7169, 10.3076) knots 0 0 0 1 2 2 2
  point P0 (30.7841, 0)
  constraints: 4 other
extrude "Extrusão10" cut sketch "Esboço11" against normal blind 0.8
sketch "Esboço12" plane through (0, 2, 0) normal (0, 1, 0) x (1, 0, 0)
  circle A0 centre (36.4205, 21.7841) radius 0.8
  line L0 (42.4205, 27.7841) -> (-59.5795, 27.7841) projected
  line L1 (42.4205, -24.2159) -> (42.4205, 27.7841) projected
  circle A1 centre (36.4205, -18.2159) radius 0.8
  circle A2 centre (-53.5795, -18.2159) radius 0.8
  circle A3 centre (-53.5795, 21.7841) radius 0.8
  line L2 (-59.5795, -24.2159) -> (42.4205, -24.2159) projected
  line L3 (-59.5795, 27.7841) -> (-59.5795, -24.2159) projected
  circle A4 centre (-53.5795, 21.7841) radius 2
  circle A5 centre (-53.5795, -18.2159) radius 2
  circle A6 centre (36.4205, 21.7841) radius 2
  circle A7 centre (36.4205, -18.2159) radius 2
  point P0 (0, 0)
  dimension "d60" = 1.6
  dimension "d61" = 6
  dimension "d62" = 6
  dimension "d63" = 1.6
  dimension "d64" = 1.6
  dimension "d65" = 1.6
  dimension "d66" = 6
  dimension "d67" = 6
  dimension "d68" = 6
  dimension "d69" = 6
  dimension "d70" = 6
  dimension "d71" = 6
  dimension "d72" = 4
  dimension "d73" = 4
  dimension "d74" = 4
  dimension "d75" = 4
  constraints: 8 centre point, 4 coincident
  measures "d60" diameter of A0
  measures "d61" distance from line of L0 A0.centre
  measures "d62" distance from line of L1 A0.centre
  measures "d63" diameter of A1
  measures "d64" diameter of A2
  measures "d65" diameter of A3
  measures "d66" distance from line of L1 A1.centre
  measures "d67" distance from line of L2 A1.centre
  measures "d68" distance from line of L2 A2.centre
  measures "d69" distance from line of L3 A2.centre
  measures "d70" distance from line of L3 A3.centre
  measures "d71" distance from line of L0 A3.centre
  measures "d72" diameter of A4
  measures "d73" diameter of A5
  measures "d74" diameter of A6
  measures "d75" diameter of A7
extrude "Extrusão12" add sketch "Esboço12" along normal blind 2.5 contours A4 | A5 | A6 | A7
sketch "Esboço13" plane through (0, 29.5, 0) normal (0, 1, 0) x (1, 0, 0)
  line L0 (43.9205, -25.7159) -> (-61.0795, -25.7159) projected
  line L1 (43.9205, -25.7159) -> (41.0355, -25.7159)
  line L2 (43.9205, 29.2841) -> (43.9205, -25.7159) projected
  line L3 (43.9205, -22.2386) -> (43.9205, -25.7159)
  line L4 (41.0355, -25.7159) -> (43.9205, -22.2386)
  line L5 (-61.0795, 29.2841) -> (43.9205, 29.2841) projected
  line L6 (43.9205, 29.2841) -> (43.9205, 25.8421)
  line L7 (43.9205, 25.8421) -> (41.0355, 29.2841)
  line L8 (41.0355, 29.2841) -> (43.9205, 29.2841)
  line L9 (-61.0795, -25.7159) -> (-61.0795, 29.2841) projected
  line L10 (-61.0795, -25.7159) -> (-58.6121, -25.7159)
  line L11 (-58.6121, -25.7159) -> (-61.0795, -23.6688)
  line L12 (-61.0795, -23.6688) -> (-61.0795, -25.7159)
  line L13 (-61.0795, 25.8421) -> (-56.9729, 29.2841)
  line L14 (-56.9729, 29.2841) -> (-61.0795, 29.2841)
  point P0 (0, 0)
  constraints: 22 end point, 8 point on line, 5 perpendicular
extrude "Extrusão13" add sketch "Esboço13" along normal blind 2 contours L0 L4 L2 | L0 L9 L11 | L7 L5 L2 | L9 L5 L13
